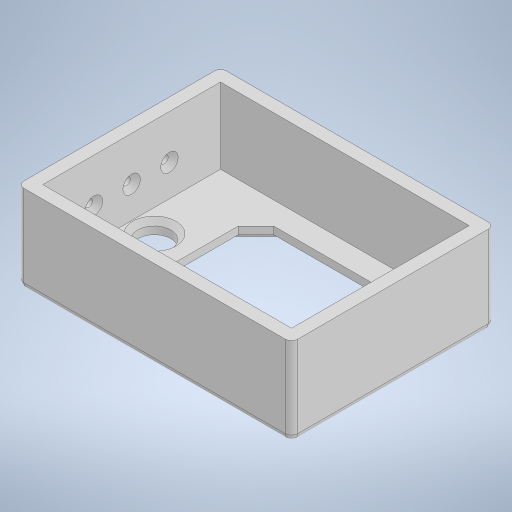
# Autodesk Inventor part: housing_top
Saved by Autodesk Inventor 2024 (Build 280153000, 153)
## iProperties
Created: 2024-03-11
Part Number: housing_top
Material: 일반
Document SubType Name: Modeling
Designer: SSAFY
Density: 1 g/cm^3
Appearance: 기본값
Author: SSAFY
Autodesk Inventor part; units mm, degrees
ref_plane "YZ Plane" through (0, 0, 0) normal (1, 0, 0) x (0, 1, 0)
ref_plane "XZ Plane" through (0, 0, 0) normal (0, 1, 0) x (-1, 0, 0)
ref_plane "XY Plane" through (0, 0, 0) normal (0, 0, 1) x (1, 0, 0)
sketch "스케치2" plane through (0, 0, 0) normal (0, 1, 0) x (-1, 0, 0)
  line L0 (49.375, -35.275) -> (-49.375, -35.275)
  line L1 (-49.375, -35.275) -> (-49.375, 35.275)
  line L2 (-49.375, 35.275) -> (49.375, 35.275)
  line L3 (49.375, 35.275) -> (49.375, -35.275)
  line L4 (49.375, -35.275) -> (-49.375, 35.275) construction
  line L5 (-49.375, -35.275) -> (49.375, 35.275) construction
  line L6 (54.375, -40.275) -> (-54.375, -40.275)
  line L7 (-54.375, -40.275) -> (-54.375, 40.275)
  line L8 (-54.375, 40.275) -> (54.375, 40.275)
  line L9 (54.375, 40.275) -> (54.375, -40.275)
  point P0 (0, 0)
  dimension "d0" = 98.75
  dimension "d1" = 70.55
  dimension "d2" = 5
  constraints: 20 end point, 4 parallel, 2 midpoint, 2 perpendicular, 1 horizontal, 3 other
  measures "d0" distance of L1.end L2.end
  measures "d1" distance of L2.end L0.start
  measures "d2" distance between parallel lines of L3 L9
extrude "돌출1" add sketch "스케치2" along normal blind 30
sketch "스케치3" plane through (0, 0, 0) normal (0, 1, 0) x (-1, 0, 0)
  line L0 (54.375, 40.275) -> (-54.375, 40.275) construction
  line L1 (54.375, -40.275) -> (-54.375, -40.275)
  line L2 (-54.375, -40.275) -> (-54.375, 40.275)
  line L3 (-54.375, 40.275) -> (54.375, 40.275)
  line L4 (54.375, 40.275) -> (54.375, -40.275)
  line L5 (54.375, -40.275) -> (-54.375, 40.275) construction
  line L6 (-54.375, -40.275) -> (54.375, 40.275) construction
  point P0 (0, 0)
  constraints: 12 end point, 2 midpoint, 2 parallel, 1 horizontal, 1 perpendicular
extrude "돌출2" add sketch "스케치3" against normal blind 5
sketch "스케치4" plane through (0, -5, 0) normal (0, -1, 0) x (1, 0, 0)
  line L0 (26.325, -26.325) -> (-26.325, -26.325)
  line L1 (-26.325, -26.325) -> (-26.325, 26.325)
  line L2 (-26.325, 26.325) -> (26.325, 26.325)
  line L3 (26.325, 26.325) -> (26.325, -26.325)
  line L4 (26.325, -26.325) -> (-26.325, 26.325) construction
  line L5 (-26.325, -26.325) -> (26.325, 26.325) construction
  line L6 (-26.325, 19.2539) -> (-19.2539, 26.325)
  line L7 (-19.2539, -26.325) -> (-26.325, -19.2539)
  line L8 (26.325, -19.2539) -> (19.2539, -26.325)
  line L9 (19.2539, 26.325) -> (26.325, 19.2539)
  point P0 (0, 0)
  dimension "d7" = 52.65
  dimension "d8" = 52.65
  dimension "d9" = 45
  dimension "d10" = 5
  dimension "d13" = 360
  constraints: 20 end point, 2 midpoint, 2 parallel, 2 point on line, 1 horizontal, 1 perpendicular, 13 other
  measures "d7" distance of L1.end L2.end
  measures "d8" distance of L2.end L0.start
  measures "d9" angle of L6 L1
  measures "d10" distance from line of L6 L1.end
extrude "돌출3" cut sketch "스케치4" against normal through all contours L0 L7 L1 L6 L2 L9 L3 L8
sketch "스케치5" plane through (-54.375, 30, -40.275) normal (-1, 0, 0) x (0, 0, 1)
  line L0 (80.55, -35) -> (0, -35) construction
  circle A0 centre (40.275, -17.5) radius 1.5
  circle A1 centre (25.275, -17.5) radius 1.5
  circle A2 centre (55.275, -17.5) radius 1.5
  point P0 (40.275, -30)
  dimension "d17" = 3
  dimension "d18" = 17.5
  dimension "d19" = 3
  dimension "d20" = 17.5
  dimension "d21" = 17.5
  dimension "d22" = 3
  dimension "d23" = 15
  dimension "d24" = 0
  dimension "d25" = 15
  constraints: 3 centre point
  measures "d17" diameter of A0
  measures "d18" distance from line of L0 A0.centre
  measures "d19" diameter of A1
  measures "d20" distance from line of L0 A1.centre
  measures "d21" distance from line of L0 A2.centre
  measures "d22" diameter of A2
  measures "d23" distance of A0.centre A1.centre
  measures "d24" horizontal distance of point (40.275, -30) A0.centre
  measures "d25" distance of A2.centre A0.centre
extrude "돌출4" cut sketch "스케치5" against normal blind 5
fillet "모깎기1" radius 2.5 8 edges at (-54.375, 12.5, 40.275) (54.375, 12.5, 40.275) (54.375, 12.5, -40.275) (-54.375, 12.5, -40.275) (-54.375, -5, 0) (0, -5, -40.275) (0, -5, 40.275) (54.375, -5, 0)
chamfer "모따기1" distance 2 angle 45 11 edges at (-49.375, 12.5, 13.5) (-49.375, 12.5, -1.5) (-49.375, 12.5, -16.5) (0, -5, -26.325) (22.7895, -5, -22.7895) (26.325, -5, 0) (22.7895, -5, 22.7895) (0, -5, 26.325) (-22.7895, -5, 22.7895) (-26.325, -5, 0) (-22.7895, -5, -22.7895)
sketch "스케치6" plane through (0, -5, 0) normal (0, -1, 0) x (1, 0, 0)
  circle A0 centre (-40.35, 0) radius 6.6
  line L0 (-54.375, 37.775) -> (-54.375, -37.775) construction
  line L1 (-26.325, -19.2539) -> (-26.325, 19.2539) construction
  point P0 (0, 0)
  dimension "d32" = 13.2
  dimension "d33" = 14.025
  dimension "d34" = 14.025
  constraints: 1 centre point
  measures "d32" diameter of A0
  measures "d33" distance from line of A0.centre L0
  measures "d34" distance from line of L1 A0.centre
extrude "돌출5" cut sketch "스케치6" against normal blind 5
chamfer "모따기2" distance 2 angle 45 1 edges at (-46.95, 0, 0)
equation "\"d33\" = d34"
